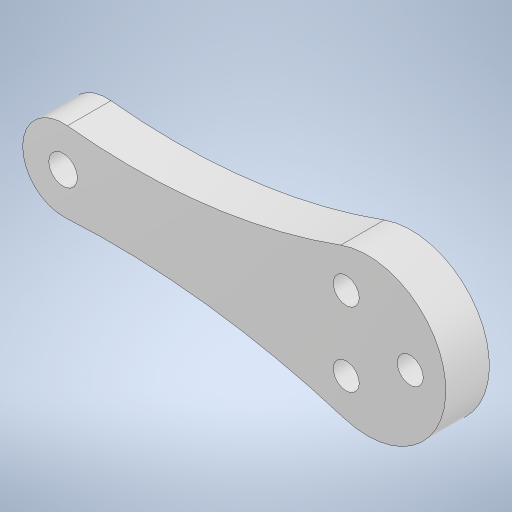
# Autodesk Inventor part: フリー節
Saved by Autodesk Inventor 2023 (Build 270158000, 158)
## iProperties
Created: 2022-04-10
Part Number: フリー節
Material: Aluminum 2014-T6
Document SubType Name: Modeling
Designer: acps
Density: 2.78927 g/cm^3
Appearance: Satin
Author: acps
Autodesk Inventor part; units mm, degrees
ref_plane "YZ Plane" through (0, 0, 0) normal (1, 0, 0) x (0, 1, 0)
ref_plane "XZ Plane" through (0, 0, 0) normal (0, 1, 0) x (-1, 0, 0)
ref_plane "XY Plane" through (0, 0, 0) normal (0, 0, 1) x (1, 0, 0)
sketch "Sketch1" plane through (0, 0, 0) normal (0, 0, 1) x (1, 0, 0)
  line L0 (52, 38.9589) -> (87, 38.9589)
  circle A0 centre (52, 38.9589) radius 1.65
  circle A1 centre (52, 38.9589) radius 4.65
  circle A2 centre (84.5463, 43.2089) radius 1.5
  circle A3 centre (84.5463, 34.7089) radius 1.5
  circle A4 centre (91.9075, 38.9589) radius 1.5
  circle A5 centre (87, 38.9589) radius 9
  arc A6 (52.4953, 43.5824) -> (83.9186, 47.4149) centre (59.9518, 113.1842) ccw
  arc A7 (84.3151, 30.3687) -> (52.2685, 34.3167) centre (57.466, -55.5331) ccw
  point P0 (0, 0)
  point P1 (0, 0)
  dimension "d2" = 35
  dimension "d3" = 3.3
  dimension "d4" = 3
  dimension "d5" = 3
  dimension "d6" = 360
  dimension "d7" = 5.5
  dimension "d8" = 18
  dimension "d9" = 70
  dimension "d10" = 90
  constraints: 8 centre point, 8 point on circle, 4 tangent, 2 coincident, 2 end point, 1 horizontal, 1 vertical alignment, 8 other
  measures "d2" distance of L0.start L0.end
  measures "d3" diameter of A0
  measures "d4" radial gap between concentric circles of A0 A1
  measures "d5" diameter of A2
  measures "d8" diameter of A5
  measures "d9" radius of A6
  measures "d10" radius of A7
extrude "Extrusion1" add sketch "Sketch1" along normal blind 5
body "Solid1"
